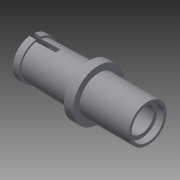
# Autodesk Inventor part: AxelDE
Saved by Autodesk Inventor 2015 (Build 190159000, 159)
## iProperties
Created: 2017-12-04
Part Number: AxelDE
Material: Generic
Document SubType Name: Modeling
Designer: Administrator
Density: 1 g/cm^3
Appearance: Default
Author: Administrator
Autodesk Inventor part; units mm, degrees
ref_plane "YZ Plane" through (0, 0, 0) normal (1, 0, 0) x (0, 1, 0)
ref_plane "XZ Plane" through (0, 0, 0) normal (0, 1, 0) x (-1, 0, 0)
ref_plane "XY Plane" through (0, 0, 0) normal (0, 0, 1) x (1, 0, 0)
sketch "Sketch1" plane through (0, 0, 0) normal (0, 0, 1) x (1, 0, 0)
  line L0 (0, 0) -> (0, 2.413)
  line L1 (0, 2.413) -> (-4.826, 2.413)
  line L2 (-4.826, 2.413) -> (-4.826, 3.175)
  line L3 (-4.826, 3.175) -> (-11.176, 3.175)
  line L4 (-11.176, 3.175) -> (-11.176, 3.81)
  line L5 (-11.176, 3.81) -> (-9.906, 3.81)
  line L6 (-9.906, 3.81) -> (-9.906, 3.429)
  line L7 (-9.906, 3.429) -> (0, 3.683)
  line L8 (0, 3.683) -> (0, 4.953)
  line L9 (0, 4.953) -> (1.778, 4.953)
  line L10 (1.778, 4.953) -> (1.778, 3.683)
  line L11 (1.778, 3.683) -> (11.43, 3.683)
  line L12 (11.43, 3.683) -> (11.43, 3.175)
  line L13 (11.43, 3.175) -> (10.16, 3.175)
  line L14 (10.16, 3.175) -> (10.16, 2.413)
  line L15 (10.16, 2.413) -> (1.778, 2.413)
  line L16 (1.778, 0) -> (0, 0)
  line L17 (1.778, 2.413) -> (1.778, 0)
  dimension "d0" = 8.382
  dimension "d2" = 0.508
  dimension "d3" = 0.762
  dimension "d4" = 1.27
  dimension "d5" = 1.778
  dimension "d6" = 2.413
  dimension "d7" = 0.254
  dimension "d8" = 1.27
  dimension "d9" = 1.27
  dimension "d10" = 1.27
  dimension "d11" = 4.826
  dimension "d12" = 6.35
  dimension "d13" = 0.635
  dimension "d15" = 0.762
  constraints: 36 end point, 12 perpendicular, 6 point on line, 1 parallel, 1 vertical
  measures "d0" distance of L14.end L15.end
  measures "d2" distance of L11.end L12.end
  measures "d3" distance of L13.end L14.end
  measures "d4" distance of L12.end L13.end
  measures "d5" distance of L8.end L9.end
  measures "d6" distance of L15.end L16.start
  measures "d7" vertical distance of L6.end L7.end
  measures "d8" distance of L4.end L5.end
  measures "d9" distance of L7.end L8.end
  measures "d10" distance of L9.end L10.end
  measures "d11" distance of L0.end L1.end
  measures "d12" distance of L2.end L3.end
  measures "d13" distance of L3.end L4.end
  measures "d15" distance of L1.end L2.end
revolve "Revolution1" add sketch "Sketch1" angle 360 about axis through (1.778, 0, 0) along (-1, 0, 0)
sketch "Sketch4" plane through (-11.176, 0, 0) normal (-1, 0, 0) x (0, 0, 1)
  line L0 (-0.508, 5.08) -> (0.508, 5.08)
  line L1 (0.508, 5.08) -> (0.508, -20.32)
  line L2 (0.508, -20.32) -> (-0.508, -20.32)
  line L3 (-0.508, -20.32) -> (-0.508, 5.08)
  point P0 (0, 0)
  point P1 (0, 4.442)
  dimension "d18" = 1.016
  dimension "d19" = 0.508
  dimension "d21" = 0
  dimension "d22" = 25.4
  constraints: 8 end point, 2 parallel, 1 horizontal, 1 perpendicular
  measures "d18" distance of L0.start L0.end
  measures "d19" distance from line of L1 point (0, 4.442)
  measures "d21" horizontal distance of point (0, 0) point (0, 4.442)
  measures "d22" distance of L0.end L1.end
extrude "Extrusion1" cut sketch "Sketch4" against normal blind 5.08
body "Solid1"
